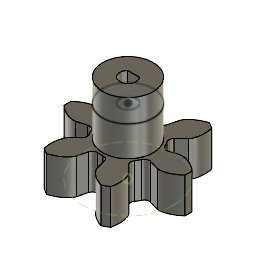
Motor Loading Gear (Autodesk Fusion 360 design; units mm, degrees)
part number: 2026-03-27-15-46-47-393
Autodesk Fusion 360 part; units mm, degrees
note: some values were not read from the file. Set by a fixed rule: which sketch regions a step uses.
(part 1 of 2)
sketch "Base Circle" plane through (0, 0, 0) normal (0, 0, 1) x (1, 0, 0)
  circle A0 centre (0, 0) radius 5.529
  circle A1 centre (0, 0) radius 1.75
  dimension "d28" = 3.5
  measures "d28" diameter of A1
extrude "Extrude1" add sketch "Base Circle" along normal blind 7 makes body 1
sketch "Gear Tooth" plane through (0, 0, 0) normal (0, 0, 1) x (1, 0, 0)
  spline S0 degree 5 poles (8.1355, -2.3104) (8.146, -2.3134) (8.1669, -2.3188) (8.1987, -2.3257) (8.2415, -2.3322) (8.2956, -2.3368) (8.3503, -2.3389) (8.4053, -2.3395) (8.4604, -2.3392) (8.5157, -2.3384) (8.5711, -2.3369) (8.6267, -2.3345) (8.6824, -2.3309) (8.7383, -2.3259) (8.7943, -2.3197) (8.8505, -2.3123) (8.9068, -2.3039) (8.9632, -2.2946) (9.0196, -2.2845) (9.0761, -2.2737) (9.1326, -2.2622) (9.1892, -2.2498) (9.2457, -2.2365) (9.3024, -2.2224) (9.359, -2.2074) (9.4157, -2.1917) (9.4723, -2.1751) (9.529, -2.1578) (9.5856, -2.1398) (9.6422, -2.1211) (9.6988, -2.1016) (9.7554, -2.0815) (9.8119, -2.0606) (9.8683, -2.0389) (9.9248, -2.0166) (9.9811, -1.9936) (10.0374, -1.9699) (10.0936, -1.9455) (10.1498, -1.9205) (10.2059, -1.8948) (10.2618, -1.8684) (10.3177, -1.8414) (10.3735, -1.8138) (10.4292, -1.7855) (10.4848, -1.7565) (10.5403, -1.7269) (10.5957, -1.6967) (10.6509, -1.6659) (10.706, -1.6345) (10.761, -1.6024) (10.8158, -1.5697) (10.8706, -1.5365) (10.9251, -1.5026) (10.9795, -1.4681) (11.0338, -1.4331) (11.0879, -1.3974) (11.1418, -1.3612) (11.1956, -1.3244) (11.2492, -1.287) (11.3026, -1.249) (11.3559, -1.2105) (11.4089, -1.1714) (11.4618, -1.1317) (11.5145, -1.0915) (11.567, -1.0507) (11.6193, -1.0094) (11.6713, -0.9676) (11.7232, -0.9251) (11.7749, -0.8822) (11.8263, -0.8387) (11.8775, -0.7947) (11.9183, -0.7591) (11.9488, -0.7321) (11.9691, -0.714) (11.9793, -0.705) knots 0 0 0 0 0 0 0.01428571 0.02857143 0.04285714 0.05714286 0.07142857 0.08571429 0.1 0.11428571 0.12857143 0.14285714 0.15714286 0.17142857 0.18571429 0.2 0.21428571 0.22857143 0.24285714 0.25714286 0.27142857 0.28571429 0.3 0.31428571 0.32857143 0.34285714 0.35714286 0.37142857 0.38571429 0.4 0.41428571 0.42857143 0.44285714 0.45714286 0.47142857 0.48571429 0.5 0.51428571 0.52857143 0.54285714 0.55714286 0.57142857 0.58571429 0.6 0.61428571 0.62857143 0.64285714 0.65714286 0.67142857 0.68571429 0.7 0.71428571 0.72857143 0.74285714 0.75714286 0.77142857 0.78571429 0.8 0.81428571 0.82857143 0.84285714 0.85714286 0.87142857 0.88571429 0.9 0.91428571 0.92857143 0.94285714 0.95714286 0.97142857 0.98571429 1 1 1 1 1 1
  spline S1 degree 5 poles (8.1355, 2.3104) (8.146, 2.3134) (8.1669, 2.3188) (8.1987, 2.3257) (8.2415, 2.3322) (8.2956, 2.3368) (8.3503, 2.3389) (8.4053, 2.3395) (8.4604, 2.3392) (8.5157, 2.3384) (8.5711, 2.3369) (8.6267, 2.3345) (8.6824, 2.3309) (8.7383, 2.3259) (8.7943, 2.3197) (8.8505, 2.3123) (8.9068, 2.3039) (8.9632, 2.2946) (9.0196, 2.2845) (9.0761, 2.2737) (9.1326, 2.2622) (9.1892, 2.2498) (9.2457, 2.2365) (9.3024, 2.2224) (9.359, 2.2074) (9.4157, 2.1917) (9.4723, 2.1751) (9.529, 2.1578) (9.5856, 2.1398) (9.6422, 2.1211) (9.6988, 2.1016) (9.7554, 2.0815) (9.8119, 2.0606) (9.8683, 2.0389) (9.9248, 2.0166) (9.9811, 1.9936) (10.0374, 1.9699) (10.0936, 1.9455) (10.1498, 1.9205) (10.2059, 1.8948) (10.2618, 1.8684) (10.3177, 1.8414) (10.3735, 1.8138) (10.4292, 1.7855) (10.4848, 1.7565) (10.5403, 1.7269) (10.5957, 1.6967) (10.6509, 1.6659) (10.706, 1.6345) (10.761, 1.6024) (10.8158, 1.5697) (10.8706, 1.5365) (10.9251, 1.5026) (10.9795, 1.4681) (11.0338, 1.4331) (11.0879, 1.3974) (11.1418, 1.3612) (11.1956, 1.3244) (11.2492, 1.287) (11.3026, 1.249) (11.3559, 1.2105) (11.4089, 1.1714) (11.4618, 1.1317) (11.5145, 1.0915) (11.567, 1.0507) (11.6193, 1.0094) (11.6713, 0.9676) (11.7232, 0.9251) (11.7749, 0.8822) (11.8263, 0.8387) (11.8775, 0.7947) (11.9183, 0.7591) (11.9488, 0.7321) (11.9691, 0.714) (11.9793, 0.705) knots 0 0 0 0 0 0 0.01428571 0.02857143 0.04285714 0.05714286 0.07142857 0.08571429 0.1 0.11428571 0.12857143 0.14285714 0.15714286 0.17142857 0.18571429 0.2 0.21428571 0.22857143 0.24285714 0.25714286 0.27142857 0.28571429 0.3 0.31428571 0.32857143 0.34285714 0.35714286 0.37142857 0.38571429 0.4 0.41428571 0.42857143 0.44285714 0.45714286 0.47142857 0.48571429 0.5 0.51428571 0.52857143 0.54285714 0.55714286 0.57142857 0.58571429 0.6 0.61428571 0.62857143 0.64285714 0.65714286 0.67142857 0.68571429 0.7 0.71428571 0.72857143 0.74285714 0.75714286 0.77142857 0.78571429 0.8 0.81428571 0.82857143 0.84285714 0.85714286 0.87142857 0.88571429 0.9 0.91428571 0.92857143 0.94285714 0.95714286 0.97142857 0.98571429 1 1 1 1 1 1
  arc A0 (11.9793, -0.705) -> (11.9793, 0.705) centre (0, 0) ccw
  line L0 (5.3091, -1.5077) -> (8.1355, -2.3104)
  line L1 (5.3091, 1.5077) -> (8.1355, 2.3104)
  line L2 (5.3091, -1.5077) -> (5.3091, 1.5077)
  point P0 (8.3903, -2.3392)
  point P1 (8.6545, -2.3325)
  point P2 (8.9246, -2.3008)
  point P3 (9.1989, -2.2473)
  point P4 (9.4764, -2.1737)
  point P5 (9.7561, -2.081)
  point P6 (10.0371, -1.9699)
  point P7 (10.3188, -1.8408)
  point P8 (10.6002, -1.694)
  point P9 (10.8807, -1.53)
  point P10 (11.1596, -1.3489)
  point P11 (11.4361, -1.1509)
  point P12 (11.7096, -0.9362)
  point P13 (8.3903, 2.3392)
  point P14 (8.6545, 2.3325)
  point P15 (8.9246, 2.3008)
  point P16 (9.1989, 2.2473)
  point P17 (9.4764, 2.1737)
  point P18 (9.7561, 2.081)
  point P19 (10.0371, 1.9699)
  point P20 (10.3188, 1.8408)
  point P21 (10.6002, 1.694)
  point P22 (10.8807, 1.53)
  point P23 (11.1596, 1.3489)
  point P24 (11.4361, 1.1509)
  point P25 (11.7096, 0.9362)
extrude "Extrude2" add sketch "Gear Tooth" along normal blind 7 bodies 1
fillet "Fillet1" radius 1 2 edges at (5.3187, -1.5104, 3.5) (5.3187, 1.5104, 3.5) on bodies 1
pattern_circular "C-Pattern1" count 6 over 360 about axis through (0, 0, 0) along (0, 0, 1) of "Extrude2", "Fillet1"
sketch "Diametrial Pitch Circle" plane through (0, 0, 0) normal (0, 0, 1) x (1, 0, 0)
  circle A0 centre (0, 0) radius 9 construction
sketch "Sketch4" plane through (0, 0, 7) normal (0, 0, 1) x (-1, 0, 0)
  arc A0 (-4.5104, 3.1978) -> (-5.0246, 2.3072) centre (0, 0) ccw
  arc A1 (-6.2065, 1.7626) -> (-5.0246, 2.3072) centre (-5.9334, 2.7245) ccw
  line L0 (-6.2065, 1.7626) -> (-8.1355, 2.3104)
  line L1 (-8.1355, -2.3104) -> (-6.2065, -1.7626)
  arc A2 (-5.0246, -2.3072) -> (-6.2065, -1.7626) centre (-5.9334, -2.7245) ccw
  line L2 (-4.6297, -4.4937) -> (-6.0686, -5.8904)
  line L3 (-2.0669, -8.2008) -> (-1.5768, -6.2563)
  line L4 (1.5768, -6.2563) -> (2.0669, -8.2008)
  line L5 (6.0686, -5.8904) -> (4.6297, -4.4937)
  line L6 (6.2065, -1.7626) -> (8.1355, -2.3104)
  line L7 (8.1355, 2.3104) -> (6.2065, 1.7626)
  line L8 (4.6297, 4.4937) -> (6.0686, 5.8904)
  line L9 (2.0669, 8.2008) -> (1.5768, 6.2563)
  line L10 (-1.5768, 6.2563) -> (-2.0669, 8.2008)
  line L11 (-6.0686, 5.8904) -> (-4.6297, 4.4937)
  circle A3 centre (0, 0) radius 1.75
  circle A4 centre (0, 0) radius 3.5
  circle A5 centre (0, 0) radius 5
  arc A6 (-4.6297, -4.4937) -> (-4.5104, -3.1978) centre (-5.3262, -3.7762) ccw
  arc A7 (-0.5142, -5.505) -> (-1.5768, -6.2563) centre (-0.6071, -6.5007) ccw
  arc A8 (1.5768, -6.2563) -> (0.5142, -5.505) centre (0.6071, -6.5007) ccw
  arc A9 (4.5104, -3.1978) -> (4.6297, -4.4937) centre (5.3262, -3.7762) ccw
  arc A10 (6.2065, -1.7626) -> (5.0246, -2.3072) centre (5.9334, -2.7245) ccw
  arc A11 (5.0246, 2.3072) -> (6.2065, 1.7626) centre (5.9334, 2.7245) ccw
  arc A12 (4.6297, 4.4937) -> (4.5104, 3.1978) centre (5.3262, 3.7762) ccw
  arc A13 (0.5142, 5.505) -> (1.5768, 6.2563) centre (0.6071, 6.5007) ccw
  arc A14 (-1.5768, 6.2563) -> (-0.5142, 5.505) centre (-0.6071, 6.5007) ccw
  arc A15 (-4.5104, 3.1978) -> (-4.6297, 4.4937) centre (-5.3262, 3.7762) ccw
  spline S0 degree 5 poles (-8.1355, 2.3104) (-8.146, 2.3134) (-8.1669, 2.3188) (-8.1987, 2.3257) (-8.2415, 2.3322) (-8.2956, 2.3368) (-8.3503, 2.3389) (-8.4053, 2.3395) (-8.4604, 2.3392) (-8.5157, 2.3384) (-8.5711, 2.3369) (-8.6267, 2.3345) (-8.6824, 2.3309) (-8.7383, 2.3259) (-8.7943, 2.3197) (-8.8505, 2.3123) (-8.9068, 2.3039) (-8.9632, 2.2946) (-9.0196, 2.2845) (-9.0761, 2.2737) (-9.1326, 2.2622) (-9.1892, 2.2498) (-9.2457, 2.2365) (-9.3024, 2.2224) (-9.359, 2.2074) (-9.4157, 2.1917) (-9.4723, 2.1751) (-9.529, 2.1578) (-9.5856, 2.1398) (-9.6422, 2.1211) (-9.6988, 2.1016) (-9.7554, 2.0815) (-9.8119, 2.0606) (-9.8683, 2.0389) (-9.9248, 2.0166) (-9.9811, 1.9936) (-10.0374, 1.9699) (-10.0936, 1.9455) (-10.1498, 1.9205) (-10.2059, 1.8948) (-10.2618, 1.8684) (-10.3177, 1.8414) (-10.3735, 1.8138) (-10.4292, 1.7855) (-10.4848, 1.7565) (-10.5403, 1.7269) (-10.5957, 1.6967) (-10.6509, 1.6659) (-10.706, 1.6345) (-10.761, 1.6024) (-10.8158, 1.5697) (-10.8706, 1.5365) (-10.9251, 1.5026) (-10.9795, 1.4681) (-11.0338, 1.4331) (-11.0879, 1.3974) (-11.1418, 1.3612) (-11.1956, 1.3244) (-11.2492, 1.287) (-11.3026, 1.249) (-11.3559, 1.2105) (-11.4089, 1.1714) (-11.4618, 1.1317) (-11.5145, 1.0915) (-11.567, 1.0507) (-11.6193, 1.0094) (-11.6713, 0.9676) (-11.7232, 0.9251) (-11.7749, 0.8822) (-11.8263, 0.8387) (-11.8775, 0.7947) (-11.9183, 0.7591) (-11.9488, 0.7321) (-11.9691, 0.714) (-11.9793, 0.705) knots 0 0 0 0 0 0 0.01428571 0.02857143 0.04285714 0.05714286 0.07142857 0.08571429 0.1 0.11428571 0.12857143 0.14285714 0.15714286 0.17142857 0.18571429 0.2 0.21428571 0.22857143 0.24285714 0.25714286 0.27142857 0.28571429 0.3 0.31428571 0.32857143 0.34285714 0.35714286 0.37142857 0.38571429 0.4 0.41428571 0.42857143 0.44285714 0.45714286 0.47142857 0.48571429 0.5 0.51428571 0.52857143 0.54285714 0.55714286 0.57142857 0.58571429 0.6 0.61428571 0.62857143 0.64285714 0.65714286 0.67142857 0.68571429 0.7 0.71428571 0.72857143 0.74285714 0.75714286 0.77142857 0.78571429 0.8 0.81428571 0.82857143 0.84285714 0.85714286 0.87142857 0.88571429 0.9 0.91428571 0.92857143 0.94285714 0.95714286 0.97142857 0.98571429 1 1 1 1 1 1
  arc A16 (-11.9793, 0.705) -> (-11.9793, -0.705) centre (0, 0) ccw
  spline S1 degree 5 poles (-11.9793, -0.705) (-11.9691, -0.714) (-11.9488, -0.7321) (-11.9183, -0.7591) (-11.8775, -0.7947) (-11.8263, -0.8387) (-11.7749, -0.8822) (-11.7232, -0.9251) (-11.6713, -0.9676) (-11.6193, -1.0094) (-11.567, -1.0507) (-11.5145, -1.0915) (-11.4618, -1.1317) (-11.4089, -1.1714) (-11.3559, -1.2105) (-11.3026, -1.249) (-11.2492, -1.287) (-11.1956, -1.3244) (-11.1418, -1.3612) (-11.0879, -1.3974) (-11.0338, -1.4331) (-10.9795, -1.4681) (-10.9251, -1.5026) (-10.8706, -1.5365) (-10.8158, -1.5697) (-10.761, -1.6024) (-10.706, -1.6345) (-10.6509, -1.6659) (-10.5957, -1.6967) (-10.5403, -1.7269) (-10.4848, -1.7565) (-10.4292, -1.7855) (-10.3735, -1.8138) (-10.3177, -1.8414) (-10.2618, -1.8684) (-10.2059, -1.8948) (-10.1498, -1.9205) (-10.0936, -1.9455) (-10.0374, -1.9699) (-9.9811, -1.9936) (-9.9248, -2.0166) (-9.8683, -2.0389) (-9.8119, -2.0606) (-9.7554, -2.0815) (-9.6988, -2.1016) (-9.6422, -2.1211) (-9.5856, -2.1398) (-9.529, -2.1578) (-9.4723, -2.1751) (-9.4157, -2.1917) (-9.359, -2.2074) (-9.3024, -2.2224) (-9.2457, -2.2365) (-9.1892, -2.2498) (-9.1326, -2.2622) (-9.0761, -2.2737) (-9.0196, -2.2845) (-8.9632, -2.2946) (-8.9068, -2.3039) (-8.8505, -2.3123) (-8.7943, -2.3197) (-8.7383, -2.3259) (-8.6824, -2.3309) (-8.6267, -2.3345) (-8.5711, -2.3369) (-8.5157, -2.3384) (-8.4604, -2.3392) (-8.4053, -2.3395) (-8.3503, -2.3389) (-8.2956, -2.3368) (-8.2415, -2.3322) (-8.1987, -2.3257) (-8.1669, -2.3188) (-8.146, -2.3134) (-8.1355, -2.3104) knots -1 -1 -1 -1 -1 -1 -0.98571429 -0.97142857 -0.95714286 -0.94285714 -0.92857143 -0.91428571 -0.9 -0.88571429 -0.87142857 -0.85714286 -0.84285714 -0.82857143 -0.81428571 -0.8 -0.78571429 -0.77142857 -0.75714286 -0.74285714 -0.72857143 -0.71428571 -0.7 -0.68571429 -0.67142857 -0.65714286 -0.64285714 -0.62857143 -0.61428571 -0.6 -0.58571429 -0.57142857 -0.55714286 -0.54285714 -0.52857143 -0.51428571 -0.5 -0.48571429 -0.47142857 -0.45714286 -0.44285714 -0.42857143 -0.41428571 -0.4 -0.38571429 -0.37142857 -0.35714286 -0.34285714 -0.32857143 -0.31428571 -0.3 -0.28571429 -0.27142857 -0.25714286 -0.24285714 -0.22857143 -0.21428571 -0.2 -0.18571429 -0.17142857 -0.15714286 -0.14285714 -0.12857143 -0.11428571 -0.1 -0.08571429 -0.07142857 -0.05714286 -0.04285714 -0.02857143 -0.01428571 0 0 0 0 0 0
  arc A17 (-5.0246, -2.3072) -> (-4.5104, -3.1978) centre (0, 0) ccw
  spline S2 degree 5 poles (-6.0686, -5.8904) (-6.0764, -5.8979) (-6.0916, -5.9134) (-6.1134, -5.9374) (-6.1405, -5.9712) (-6.1715, -6.0158) (-6.2007, -6.0621) (-6.2287, -6.1095) (-6.2561, -6.1573) (-6.283, -6.2056) (-6.3094, -6.2544) (-6.3351, -6.3037) (-6.3598, -6.3537) (-6.3835, -6.4046) (-6.4061, -6.4563) (-6.4278, -6.5086) (-6.4486, -6.5616) (-6.4688, -6.6151) (-6.4883, -6.669) (-6.5072, -6.7233) (-6.5254, -6.778) (-6.5429, -6.8332) (-6.5597, -6.8888) (-6.5758, -6.9449) (-6.5912, -7.0014) (-6.6059, -7.0584) (-6.6199, -7.1157) (-6.6332, -7.1734) (-6.6459, -7.2315) (-6.658, -7.2899) (-6.6695, -7.3486) (-6.6803, -7.4077) (-6.6904, -7.467) (-6.6999, -7.5268) (-6.7088, -7.5868) (-6.7171, -7.6471) (-6.7247, -7.7077) (-6.7317, -7.7686) (-6.7381, -7.8297) (-6.7439, -7.8911) (-6.749, -7.9528) (-6.7536, -8.0147) (-6.7575, -8.0769) (-6.7609, -8.1392) (-6.7636, -8.2019) (-6.7657, -8.2647) (-6.7672, -8.3277) (-6.7682, -8.391) (-6.7685, -8.4545) (-6.7682, -8.5181) (-6.7674, -8.5819) (-6.7659, -8.6459) (-6.7638, -8.7101) (-6.7612, -8.7745) (-6.758, -8.839) (-6.7541, -8.9037) (-6.7497, -8.9685) (-6.7447, -9.0335) (-6.7391, -9.0986) (-6.733, -9.1639) (-6.7262, -9.2292) (-6.7189, -9.2947) (-6.711, -9.3604) (-6.7025, -9.4261) (-6.6935, -9.4919) (-6.6838, -9.5579) (-6.6736, -9.6239) (-6.6628, -9.69) (-6.6514, -9.7562) (-6.6395, -9.8225) (-6.627, -9.8889) (-6.6165, -9.942) (-6.6084, -9.9819) (-6.6029, -10.0086) (-6.6001, -10.0219) knots 0 0 0 0 0 0 0.01428571 0.02857143 0.04285714 0.05714286 0.07142857 0.08571429 0.1 0.11428571 0.12857143 0.14285714 0.15714286 0.17142857 0.18571429 0.2 0.21428571 0.22857143 0.24285714 0.25714286 0.27142857 0.28571429 0.3 0.31428571 0.32857143 0.34285714 0.35714286 0.37142857 0.38571429 0.4 0.41428571 0.42857143 0.44285714 0.45714286 0.47142857 0.48571429 0.5 0.51428571 0.52857143 0.54285714 0.55714286 0.57142857 0.58571429 0.6 0.61428571 0.62857143 0.64285714 0.65714286 0.67142857 0.68571429 0.7 0.71428571 0.72857143 0.74285714 0.75714286 0.77142857 0.78571429 0.8 0.81428571 0.82857143 0.84285714 0.85714286 0.87142857 0.88571429 0.9 0.91428571 0.92857143 0.94285714 0.95714286 0.97142857 0.98571429 1 1 1 1 1 1
  arc A18 (-6.6001, -10.0219) -> (-5.3791, -10.7268) centre (0, 0) ccw
  spline S3 degree 5 poles (-5.3791, -10.7268) (-5.3662, -10.7226) (-5.3404, -10.7141) (-5.3018, -10.7011) (-5.2505, -10.6836) (-5.1868, -10.6612) (-5.1234, -10.6384) (-5.0604, -10.6152) (-4.9977, -10.5915) (-4.9354, -10.5673) (-4.8735, -10.5427) (-4.812, -10.5176) (-4.7508, -10.4921) (-4.69, -10.4661) (-4.6296, -10.4397) (-4.5696, -10.4129) (-4.5101, -10.3856) (-4.4509, -10.3578) (-4.3921, -10.3297) (-4.3338, -10.3011) (-4.2758, -10.2721) (-4.2183, -10.2426) (-4.1613, -10.2127) (-4.1047, -10.1824) (-4.0485, -10.1517) (-3.9928, -10.1205) (-3.9375, -10.0889) (-3.8827, -10.0569) (-3.8284, -10.0245) (-3.7746, -9.9916) (-3.7212, -9.9584) (-3.6684, -9.9247) (-3.616, -9.8906) (-3.5641, -9.8561) (-3.5128, -9.8212) (-3.462, -9.7859) (-3.4117, -9.7502) (-3.3619, -9.7141) (-3.3127, -9.6776) (-3.264, -9.6407) (-3.2159, -9.6034) (-3.1684, -9.5657) (-3.1214, -9.5276) (-3.0751, -9.4891) (-3.0293, -9.4502) (-2.9842, -9.4109) (-2.9397, -9.3713) (-2.8958, -9.3312) (-2.8525, -9.2908) (-2.8098, -9.25) (-2.7678, -9.2089) (-2.7265, -9.1673) (-2.686, -9.1253) (-2.6462, -9.0829) (-2.6072, -9.0401) (-2.5689, -8.997) (-2.5313, -8.9535) (-2.4944, -8.9097) (-2.4582, -8.8655) (-2.4228, -8.8209) (-2.3882, -8.776) (-2.3548, -8.7305) (-2.3226, -8.6846) (-2.2916, -8.6382) (-2.2617, -8.5913) (-2.2327, -8.544) (-2.2044, -8.4966) (-2.1766, -8.4489) (-2.1496, -8.401) (-2.1241, -8.3526) (-2.101, -8.3034) (-2.0852, -8.2631) (-2.0753, -8.2322) (-2.0696, -8.2113) (-2.0669, -8.2008) knots -1 -1 -1 -1 -1 -1 -0.98571429 -0.97142857 -0.95714286 -0.94285714 -0.92857143 -0.91428571 -0.9 -0.88571429 -0.87142857 -0.85714286 -0.84285714 -0.82857143 -0.81428571 -0.8 -0.78571429 -0.77142857 -0.75714286 -0.74285714 -0.72857143 -0.71428571 -0.7 -0.68571429 -0.67142857 -0.65714286 -0.64285714 -0.62857143 -0.61428571 -0.6 -0.58571429 -0.57142857 -0.55714286 -0.54285714 -0.52857143 -0.51428571 -0.5 -0.48571429 -0.47142857 -0.45714286 -0.44285714 -0.42857143 -0.41428571 -0.4 -0.38571429 -0.37142857 -0.35714286 -0.34285714 -0.32857143 -0.31428571 -0.3 -0.28571429 -0.27142857 -0.25714286 -0.24285714 -0.22857143 -0.21428571 -0.2 -0.18571429 -0.17142857 -0.15714286 -0.14285714 -0.12857143 -0.11428571 -0.1 -0.08571429 -0.07142857 -0.05714286 -0.04285714 -0.02857143 -0.01428571 0 0 0 0 0 0
  arc A19 (-0.5142, -5.505) -> (0.5142, -5.505) centre (0, 0) ccw
  spline S4 degree 5 poles (2.0669, -8.2008) (2.0696, -8.2113) (2.0753, -8.2322) (2.0852, -8.2631) (2.101, -8.3034) (2.1241, -8.3526) (2.1496, -8.401) (2.1766, -8.4489) (2.2044, -8.4966) (2.2327, -8.544) (2.2617, -8.5913) (2.2916, -8.6382) (2.3226, -8.6846) (2.3548, -8.7305) (2.3882, -8.776) (2.4228, -8.8209) (2.4582, -8.8655) (2.4944, -8.9097) (2.5313, -8.9535) (2.5689, -8.997) (2.6072, -9.0401) (2.6462, -9.0829) (2.686, -9.1253) (2.7265, -9.1673) (2.7678, -9.2089) (2.8098, -9.25) (2.8525, -9.2908) (2.8958, -9.3312) (2.9397, -9.3713) (2.9842, -9.4109) (3.0293, -9.4502) (3.0751, -9.4891) (3.1214, -9.5276) (3.1684, -9.5657) (3.2159, -9.6034) (3.264, -9.6407) (3.3127, -9.6776) (3.3619, -9.7141) (3.4117, -9.7502) (3.462, -9.7859) (3.5128, -9.8212) (3.5641, -9.8561) (3.616, -9.8906) (3.6684, -9.9247) (3.7212, -9.9584) (3.7746, -9.9916) (3.8284, -10.0245) (3.8827, -10.0569) (3.9375, -10.0889) (3.9928, -10.1205) (4.0485, -10.1517) (4.1047, -10.1824) (4.1613, -10.2127) (4.2183, -10.2426) (4.2758, -10.2721) (4.3338, -10.3011) (4.3921, -10.3297) (4.4509, -10.3578) (4.5101, -10.3856) (4.5696, -10.4129) (4.6296, -10.4397) (4.69, -10.4661) (4.7508, -10.4921) (4.812, -10.5176) (4.8735, -10.5427) (4.9354, -10.5673) (4.9977, -10.5915) (5.0604, -10.6152) (5.1234, -10.6384) (5.1868, -10.6612) (5.2505, -10.6836) (5.3018, -10.7011) (5.3404, -10.7141) (5.3662, -10.7226) (5.3791, -10.7268) knots 0 0 0 0 0 0 0.01428571 0.02857143 0.04285714 0.05714286 0.07142857 0.08571429 0.1 0.11428571 0.12857143 0.14285714 0.15714286 0.17142857 0.18571429 0.2 0.21428571 0.22857143 0.24285714 0.25714286 0.27142857 0.28571429 0.3 0.31428571 0.32857143 0.34285714 0.35714286 0.37142857 0.38571429 0.4 0.41428571 0.42857143 0.44285714 0.45714286 0.47142857 0.48571429 0.5 0.51428571 0.52857143 0.54285714 0.55714286 0.57142857 0.58571429 0.6 0.61428571 0.62857143 0.64285714 0.65714286 0.67142857 0.68571429 0.7 0.71428571 0.72857143 0.74285714 0.75714286 0.77142857 0.78571429 0.8 0.81428571 0.82857143 0.84285714 0.85714286 0.87142857 0.88571429 0.9 0.91428571 0.92857143 0.94285714 0.95714286 0.97142857 0.98571429 1 1 1 1 1 1
  arc A20 (5.3791, -10.7268) -> (6.6001, -10.0219) centre (0, 0) ccw
  spline S5 degree 5 poles (6.6001, -10.0219) (6.6029, -10.0086) (6.6084, -9.9819) (6.6165, -9.942) (6.627, -9.8889) (6.6395, -9.8225) (6.6514, -9.7562) (6.6628, -9.69) (6.6736, -9.6239) (6.6838, -9.5579) (6.6935, -9.4919) (6.7025, -9.4261) (6.711, -9.3604) (6.7189, -9.2947) (6.7262, -9.2292) (6.733, -9.1639) (6.7391, -9.0986) (6.7447, -9.0335) (6.7497, -8.9685) (6.7541, -8.9037) (6.758, -8.839) (6.7612, -8.7745) (6.7638, -8.7101) (6.7659, -8.6459) (6.7674, -8.5819) (6.7682, -8.5181) (6.7685, -8.4545) (6.7682, -8.391) (6.7672, -8.3277) (6.7657, -8.2647) (6.7636, -8.2019) (6.7609, -8.1392) (6.7575, -8.0769) (6.7536, -8.0147) (6.749, -7.9528) (6.7439, -7.8911) (6.7381, -7.8297) (6.7317, -7.7686) (6.7247, -7.7077) (6.7171, -7.6471) (6.7088, -7.5868) (6.6999, -7.5268) (6.6904, -7.467) (6.6803, -7.4077) (6.6695, -7.3486) (6.658, -7.2899) (6.6459, -7.2315) (6.6332, -7.1734) (6.6199, -7.1157) (6.6059, -7.0584) (6.5912, -7.0014) (6.5758, -6.9449) (6.5597, -6.8888) (6.5429, -6.8332) (6.5254, -6.778) (6.5072, -6.7233) (6.4883, -6.669) (6.4688, -6.6151) (6.4486, -6.5616) (6.4278, -6.5086) (6.4061, -6.4563) (6.3835, -6.4046) (6.3598, -6.3537) (6.3351, -6.3037) (6.3094, -6.2544) (6.283, -6.2056) (6.2561, -6.1573) (6.2287, -6.1095) (6.2007, -6.0621) (6.1715, -6.0158) (6.1405, -5.9712) (6.1134, -5.9374) (6.0916, -5.9134) (6.0764, -5.8979) (6.0686, -5.8904) knots -1 -1 -1 -1 -1 -1 -0.98571429 -0.97142857 -0.95714286 -0.94285714 -0.92857143 -0.91428571 -0.9 -0.88571429 -0.87142857 -0.85714286 -0.84285714 -0.82857143 -0.81428571 -0.8 -0.78571429 -0.77142857 -0.75714286 -0.74285714 -0.72857143 -0.71428571 -0.7 -0.68571429 -0.67142857 -0.65714286 -0.64285714 -0.62857143 -0.61428571 -0.6 -0.58571429 -0.57142857 -0.55714286 -0.54285714 -0.52857143 -0.51428571 -0.5 -0.48571429 -0.47142857 -0.45714286 -0.44285714 -0.42857143 -0.41428571 -0.4 -0.38571429 -0.37142857 -0.35714286 -0.34285714 -0.32857143 -0.31428571 -0.3 -0.28571429 -0.27142857 -0.25714286 -0.24285714 -0.22857143 -0.21428571 -0.2 -0.18571429 -0.17142857 -0.15714286 -0.14285714 -0.12857143 -0.11428571 -0.1 -0.08571429 -0.07142857 -0.05714286 -0.04285714 -0.02857143 -0.01428571 0 0 0 0 0 0
  arc A21 (4.5104, -3.1978) -> (5.0246, -2.3072) centre (0, 0) ccw
  spline S6 degree 5 poles (8.1355, -2.3104) (8.146, -2.3134) (8.1669, -2.3188) (8.1987, -2.3257) (8.2415, -2.3322) (8.2956, -2.3368) (8.3503, -2.3389) (8.4053, -2.3395) (8.4604, -2.3392) (8.5157, -2.3384) (8.5711, -2.3369) (8.6267, -2.3345) (8.6824, -2.3309) (8.7383, -2.3259) (8.7943, -2.3197) (8.8505, -2.3123) (8.9068, -2.3039) (8.9632, -2.2946) (9.0196, -2.2845) (9.0761, -2.2737) (9.1326, -2.2622) (9.1892, -2.2498) (9.2457, -2.2365) (9.3024, -2.2224) (9.359, -2.2074) (9.4157, -2.1917) (9.4723, -2.1751) (9.529, -2.1578) (9.5856, -2.1398) (9.6422, -2.1211) (9.6988, -2.1016) (9.7554, -2.0815) (9.8119, -2.0606) (9.8683, -2.0389) (9.9248, -2.0166) (9.9811, -1.9936) (10.0374, -1.9699) (10.0936, -1.9455) (10.1498, -1.9205) (10.2059, -1.8948) (10.2618, -1.8684) (10.3177, -1.8414) (10.3735, -1.8138) (10.4292, -1.7855) (10.4848, -1.7565) (10.5403, -1.7269) (10.5957, -1.6967) (10.6509, -1.6659) (10.706, -1.6345) (10.761, -1.6024) (10.8158, -1.5697) (10.8706, -1.5365) (10.9251, -1.5026) (10.9795, -1.4681) (11.0338, -1.4331) (11.0879, -1.3974) (11.1418, -1.3612) (11.1956, -1.3244) (11.2492, -1.287) (11.3026, -1.249) (11.3559, -1.2105) (11.4089, -1.1714) (11.4618, -1.1317) (11.5145, -1.0915) (11.567, -1.0507) (11.6193, -1.0094) (11.6713, -0.9676) (11.7232, -0.9251) (11.7749, -0.8822) (11.8263, -0.8387) (11.8775, -0.7947) (11.9183, -0.7591) (11.9488, -0.7321) (11.9691, -0.714) (11.9793, -0.705) knots 0 0 0 0 0 0 0.01428571 0.02857143 0.04285714 0.05714286 0.07142857 0.08571429 0.1 0.11428571 0.12857143 0.14285714 0.15714286 0.17142857 0.18571429 0.2 0.21428571 0.22857143 0.24285714 0.25714286 0.27142857 0.28571429 0.3 0.31428571 0.32857143 0.34285714 0.35714286 0.37142857 0.38571429 0.4 0.41428571 0.42857143 0.44285714 0.45714286 0.47142857 0.48571429 0.5 0.51428571 0.52857143 0.54285714 0.55714286 0.57142857 0.58571429 0.6 0.61428571 0.62857143 0.64285714 0.65714286 0.67142857 0.68571429 0.7 0.71428571 0.72857143 0.74285714 0.75714286 0.77142857 0.78571429 0.8 0.81428571 0.82857143 0.84285714 0.85714286 0.87142857 0.88571429 0.9 0.91428571 0.92857143 0.94285714 0.95714286 0.97142857 0.98571429 1 1 1 1 1 1
  arc A22 (11.9793, -0.705) -> (11.9793, 0.705) centre (0, 0) ccw
  spline S7 degree 5 poles (11.9793, 0.705) (11.9691, 0.714) (11.9488, 0.7321) (11.9183, 0.7591) (11.8775, 0.7947) (11.8263, 0.8387) (11.7749, 0.8822) (11.7232, 0.9251) (11.6713, 0.9676) (11.6193, 1.0094) (11.567, 1.0507) (11.5145, 1.0915) (11.4618, 1.1317) (11.4089, 1.1714) (11.3559, 1.2105) (11.3026, 1.249) (11.2492, 1.287) (11.1956, 1.3244) (11.1418, 1.3612) (11.0879, 1.3974) (11.0338, 1.4331) (10.9795, 1.4681) (10.9251, 1.5026) (10.8706, 1.5365) (10.8158, 1.5697) (10.761, 1.6024) (10.706, 1.6345) (10.6509, 1.6659) (10.5957, 1.6967) (10.5403, 1.7269) (10.4848, 1.7565) (10.4292, 1.7855) (10.3735, 1.8138) (10.3177, 1.8414) (10.2618, 1.8684) (10.2059, 1.8948) (10.1498, 1.9205) (10.0936, 1.9455) (10.0374, 1.9699) (9.9811, 1.9936) (9.9248, 2.0166) (9.8683, 2.0389) (9.8119, 2.0606) (9.7554, 2.0815) (9.6988, 2.1016) (9.6422, 2.1211) (9.5856, 2.1398) (9.529, 2.1578) (9.4723, 2.1751) (9.4157, 2.1917) (9.359, 2.2074) (9.3024, 2.2224) (9.2457, 2.2365) (9.1892, 2.2498) (9.1326, 2.2622) (9.0761, 2.2737) (9.0196, 2.2845) (8.9632, 2.2946) (8.9068, 2.3039) (8.8505, 2.3123) (8.7943, 2.3197) (8.7383, 2.3259) (8.6824, 2.3309) (8.6267, 2.3345) (8.5711, 2.3369) (8.5157, 2.3384) (8.4604, 2.3392) (8.4053, 2.3395) (8.3503, 2.3389) (8.2956, 2.3368) (8.2415, 2.3322) (8.1987, 2.3257) (8.1669, 2.3188) (8.146, 2.3134) (8.1355, 2.3104) knots -1 -1 -1 -1 -1 -1 -0.98571429 -0.97142857 -0.95714286 -0.94285714 -0.92857143 -0.91428571 -0.9 -0.88571429 -0.87142857 -0.85714286 -0.84285714 -0.82857143 -0.81428571 -0.8 -0.78571429 -0.77142857 -0.75714286 -0.74285714 -0.72857143 -0.71428571 -0.7 -0.68571429 -0.67142857 -0.65714286 -0.64285714 -0.62857143 -0.61428571 -0.6 -0.58571429 -0.57142857 -0.55714286 -0.54285714 -0.52857143 -0.51428571 -0.5 -0.48571429 -0.47142857 -0.45714286 -0.44285714 -0.42857143 -0.41428571 -0.4 -0.38571429 -0.37142857 -0.35714286 -0.34285714 -0.32857143 -0.31428571 -0.3 -0.28571429 -0.27142857 -0.25714286 -0.24285714 -0.22857143 -0.21428571 -0.2 -0.18571429 -0.17142857 -0.15714286 -0.14285714 -0.12857143 -0.11428571 -0.1 -0.08571429 -0.07142857 -0.05714286 -0.04285714 -0.02857143 -0.01428571 0 0 0 0 0 0
  arc A23 (5.0246, 2.3072) -> (4.5104, 3.1978) centre (0, 0) ccw
  spline S8 degree 5 poles (6.0686, 5.8904) (6.0764, 5.8979) (6.0916, 5.9134) (6.1134, 5.9374) (6.1405, 5.9712) (6.1715, 6.0158) (6.2007, 6.0621) (6.2287, 6.1095) (6.2561, 6.1573) (6.283, 6.2056) (6.3094, 6.2544) (6.3351, 6.3037) (6.3598, 6.3537) (6.3835, 6.4046) (6.4061, 6.4563) (6.4278, 6.5086) (6.4486, 6.5616) (6.4688, 6.6151) (6.4883, 6.669) (6.5072, 6.7233) (6.5254, 6.778) (6.5429, 6.8332) (6.5597, 6.8888) (6.5758, 6.9449) (6.5912, 7.0014) (6.6059, 7.0584) (6.6199, 7.1157) (6.6332, 7.1734) (6.6459, 7.2315) (6.658, 7.2899) (6.6695, 7.3486) (6.6803, 7.4077) (6.6904, 7.467) (6.6999, 7.5268) (6.7088, 7.5868) (6.7171, 7.6471) (6.7247, 7.7077) (6.7317, 7.7686) (6.7381, 7.8297) (6.7439, 7.8911) (6.749, 7.9528) (6.7536, 8.0147) (6.7575, 8.0769) (6.7609, 8.1392) (6.7636, 8.2019) (6.7657, 8.2647) (6.7672, 8.3277) (6.7682, 8.391) (6.7685, 8.4545) (6.7682, 8.5181) (6.7674, 8.5819) (6.7659, 8.6459) (6.7638, 8.7101) (6.7612, 8.7745) (6.758, 8.839) (6.7541, 8.9037) (6.7497, 8.9685) (6.7447, 9.0335) (6.7391, 9.0986) (6.733, 9.1639) (6.7262, 9.2292) (6.7189, 9.2947) (6.711, 9.3604) (6.7025, 9.4261) (6.6935, 9.4919) (6.6838, 9.5579) (6.6736, 9.6239) (6.6628, 9.69) (6.6514, 9.7562) (6.6395, 9.8225) (6.627, 9.8889) (6.6165, 9.942) (6.6084, 9.9819) (6.6029, 10.0086) (6.6001, 10.0219) knots 0 0 0 0 0 0 0.01428571 0.02857143 0.04285714 0.05714286 0.07142857 0.08571429 0.1 0.11428571 0.12857143 0.14285714 0.15714286 0.17142857 0.18571429 0.2 0.21428571 0.22857143 0.24285714 0.25714286 0.27142857 0.28571429 0.3 0.31428571 0.32857143 0.34285714 0.35714286 0.37142857 0.38571429 0.4 0.41428571 0.42857143 0.44285714 0.45714286 0.47142857 0.48571429 0.5 0.51428571 0.52857143 0.54285714 0.55714286 0.57142857 0.58571429 0.6 0.61428571 0.62857143 0.64285714 0.65714286 0.67142857 0.68571429 0.7 0.71428571 0.72857143 0.74285714 0.75714286 0.77142857 0.78571429 0.8 0.81428571 0.82857143 0.84285714 0.85714286 0.87142857 0.88571429 0.9 0.91428571 0.92857143 0.94285714 0.95714286 0.97142857 0.98571429 1 1 1 1 1 1
  arc A24 (6.6001, 10.0219) -> (5.3791, 10.7268) centre (0, 0) ccw
  spline S9 degree 5 poles (5.3791, 10.7268) (5.3662, 10.7226) (5.3404, 10.7141) (5.3018, 10.7011) (5.2505, 10.6836) (5.1868, 10.6612) (5.1234, 10.6384) (5.0604, 10.6152) (4.9977, 10.5915) (4.9354, 10.5673) (4.8735, 10.5427) (4.812, 10.5176) (4.7508, 10.4921) (4.69, 10.4661) (4.6296, 10.4397) (4.5696, 10.4129) (4.5101, 10.3856) (4.4509, 10.3578) (4.3921, 10.3297) (4.3338, 10.3011) (4.2758, 10.2721) (4.2183, 10.2426) (4.1613, 10.2127) (4.1047, 10.1824) (4.0485, 10.1517) (3.9928, 10.1205) (3.9375, 10.0889) (3.8827, 10.0569) (3.8284, 10.0245) (3.7746, 9.9916) (3.7212, 9.9584) (3.6684, 9.9247) (3.616, 9.8906) (3.5641, 9.8561) (3.5128, 9.8212) (3.462, 9.7859) (3.4117, 9.7502) (3.3619, 9.7141) (3.3127, 9.6776) (3.264, 9.6407) (3.2159, 9.6034) (3.1684, 9.5657) (3.1214, 9.5276) (3.0751, 9.4891) (3.0293, 9.4502) (2.9842, 9.4109) (2.9397, 9.3713) (2.8958, 9.3312) (2.8525, 9.2908) (2.8098, 9.25) (2.7678, 9.2089) (2.7265, 9.1673) (2.686, 9.1253) (2.6462, 9.0829) (2.6072, 9.0401) (2.5689, 8.997) (2.5313, 8.9535) (2.4944, 8.9097) (2.4582, 8.8655) (2.4228, 8.8209) (2.3882, 8.776) (2.3548, 8.7305) (2.3226, 8.6846) (2.2916, 8.6382) (2.2617, 8.5913) (2.2327, 8.544) (2.2044, 8.4966) (2.1766, 8.4489) (2.1496, 8.401) (2.1241, 8.3526) (2.101, 8.3034) (2.0852, 8.2631) (2.0753, 8.2322) (2.0696, 8.2113) (2.0669, 8.2008) knots -1 -1 -1 -1 -1 -1 -0.98571429 -0.97142857 -0.95714286 -0.94285714 -0.92857143 -0.91428571 -0.9 -0.88571429 -0.87142857 -0.85714286 -0.84285714 -0.82857143 -0.81428571 -0.8 -0.78571429 -0.77142857 -0.75714286 -0.74285714 -0.72857143 -0.71428571 -0.7 -0.68571429 -0.67142857 -0.65714286 -0.64285714 -0.62857143 -0.61428571 -0.6 -0.58571429 -0.57142857 -0.55714286 -0.54285714 -0.52857143 -0.51428571 -0.5 -0.48571429 -0.47142857 -0.45714286 -0.44285714 -0.42857143 -0.41428571 -0.4 -0.38571429 -0.37142857 -0.35714286 -0.34285714 -0.32857143 -0.31428571 -0.3 -0.28571429 -0.27142857 -0.25714286 -0.24285714 -0.22857143 -0.21428571 -0.2 -0.18571429 -0.17142857 -0.15714286 -0.14285714 -0.12857143 -0.11428571 -0.1 -0.08571429 -0.07142857 -0.05714286 -0.04285714 -0.02857143 -0.01428571 0 0 0 0 0 0
  arc A25 (0.5142, 5.505) -> (-0.5142, 5.505) centre (0, 0) ccw
  spline S10 degree 5 poles (-2.0669, 8.2008) (-2.0696, 8.2113) (-2.0753, 8.2322) (-2.0852, 8.2631) (-2.101, 8.3034) (-2.1241, 8.3526) (-2.1496, 8.401) (-2.1766, 8.4489) (-2.2044, 8.4966) (-2.2327, 8.544) (-2.2617, 8.5913) (-2.2916, 8.6382) (-2.3226, 8.6846) (-2.3548, 8.7305) (-2.3882, 8.776) (-2.4228, 8.8209) (-2.4582, 8.8655) (-2.4944, 8.9097) (-2.5313, 8.9535) (-2.5689, 8.997) (-2.6072, 9.0401) (-2.6462, 9.0829) (-2.686, 9.1253) (-2.7265, 9.1673) (-2.7678, 9.2089) (-2.8098, 9.25) (-2.8525, 9.2908) (-2.8958, 9.3312) (-2.9397, 9.3713) (-2.9842, 9.4109) (-3.0293, 9.4502) (-3.0751, 9.4891) (-3.1214, 9.5276) (-3.1684, 9.5657) (-3.2159, 9.6034) (-3.264, 9.6407) (-3.3127, 9.6776) (-3.3619, 9.7141) (-3.4117, 9.7502) (-3.462, 9.7859) (-3.5128, 9.8212) (-3.5641, 9.8561) (-3.616, 9.8906) (-3.6684, 9.9247) (-3.7212, 9.9584) (-3.7746, 9.9916) (-3.8284, 10.0245) (-3.8827, 10.0569) (-3.9375, 10.0889) (-3.9928, 10.1205) (-4.0485, 10.1517) (-4.1047, 10.1824) (-4.1613, 10.2127) (-4.2183, 10.2426) (-4.2758, 10.2721) (-4.3338, 10.3011) (-4.3921, 10.3297) (-4.4509, 10.3578) (-4.5101, 10.3856) (-4.5696, 10.4129) (-4.6296, 10.4397) (-4.69, 10.4661) (-4.7508, 10.4921) (-4.812, 10.5176) (-4.8735, 10.5427) (-4.9354, 10.5673) (-4.9977, 10.5915) (-5.0604, 10.6152) (-5.1234, 10.6384) (-5.1868, 10.6612) (-5.2505, 10.6836) (-5.3018, 10.7011) (-5.3404, 10.7141) (-5.3662, 10.7226) (-5.3791, 10.7268) knots 0 0 0 0 0 0 0.01428571 0.02857143 0.04285714 0.05714286 0.07142857 0.08571429 0.1 0.11428571 0.12857143 0.14285714 0.15714286 0.17142857 0.18571429 0.2 0.21428571 0.22857143 0.24285714 0.25714286 0.27142857 0.28571429 0.3 0.31428571 0.32857143 0.34285714 0.35714286 0.37142857 0.38571429 0.4 0.41428571 0.42857143 0.44285714 0.45714286 0.47142857 0.48571429 0.5 0.51428571 0.52857143 0.54285714 0.55714286 0.57142857 0.58571429 0.6 0.61428571 0.62857143 0.64285714 0.65714286 0.67142857 0.68571429 0.7 0.71428571 0.72857143 0.74285714 0.75714286 0.77142857 0.78571429 0.8 0.81428571 0.82857143 0.84285714 0.85714286 0.87142857 0.88571429 0.9 0.91428571 0.92857143 0.94285714 0.95714286 0.97142857 0.98571429 1 1 1 1 1 1
  arc A26 (-5.3791, 10.7268) -> (-6.6001, 10.0219) centre (0, 0) ccw
  spline S11 degree 5 poles (-6.6001, 10.0219) (-6.6029, 10.0086) (-6.6084, 9.9819) (-6.6165, 9.942) (-6.627, 9.8889) (-6.6395, 9.8225) (-6.6514, 9.7562) (-6.6628, 9.69) (-6.6736, 9.6239) (-6.6838, 9.5579) (-6.6935, 9.4919) (-6.7025, 9.4261) (-6.711, 9.3604) (-6.7189, 9.2947) (-6.7262, 9.2292) (-6.733, 9.1639) (-6.7391, 9.0986) (-6.7447, 9.0335) (-6.7497, 8.9685) (-6.7541, 8.9037) (-6.758, 8.839) (-6.7612, 8.7745) (-6.7638, 8.7101) (-6.7659, 8.6459) (-6.7674, 8.5819) (-6.7682, 8.5181) (-6.7685, 8.4545) (-6.7682, 8.391) (-6.7672, 8.3277) (-6.7657, 8.2647) (-6.7636, 8.2019) (-6.7609, 8.1392) (-6.7575, 8.0769) (-6.7536, 8.0147) (-6.749, 7.9528) (-6.7439, 7.8911) (-6.7381, 7.8297) (-6.7317, 7.7686) (-6.7247, 7.7077) (-6.7171, 7.6471) (-6.7088, 7.5868) (-6.6999, 7.5268) (-6.6904, 7.467) (-6.6803, 7.4077) (-6.6695, 7.3486) (-6.658, 7.2899) (-6.6459, 7.2315) (-6.6332, 7.1734) (-6.6199, 7.1157) (-6.6059, 7.0584) (-6.5912, 7.0014) (-6.5758, 6.9449) (-6.5597, 6.8888) (-6.5429, 6.8332) (-6.5254, 6.778) (-6.5072, 6.7233) (-6.4883, 6.669) (-6.4688, 6.6151) (-6.4486, 6.5616) (-6.4278, 6.5086) (-6.4061, 6.4563) (-6.3835, 6.4046) (-6.3598, 6.3537) (-6.3351, 6.3037) (-6.3094, 6.2544) (-6.283, 6.2056) (-6.2561, 6.1573) (-6.2287, 6.1095) (-6.2007, 6.0621) (-6.1715, 6.0158) (-6.1405, 5.9712) (-6.1134, 5.9374) (-6.0916, 5.9134) (-6.0764, 5.8979) (-6.0686, 5.8904) knots -1 -1 -1 -1 -1 -1 -0.98571429 -0.97142857 -0.95714286 -0.94285714 -0.92857143 -0.91428571 -0.9 -0.88571429 -0.87142857 -0.85714286 -0.84285714 -0.82857143 -0.81428571 -0.8 -0.78571429 -0.77142857 -0.75714286 -0.74285714 -0.72857143 -0.71428571 -0.7 -0.68571429 -0.67142857 -0.65714286 -0.64285714 -0.62857143 -0.61428571 -0.6 -0.58571429 -0.57142857 -0.55714286 -0.54285714 -0.52857143 -0.51428571 -0.5 -0.48571429 -0.47142857 -0.45714286 -0.44285714 -0.42857143 -0.41428571 -0.4 -0.38571429 -0.37142857 -0.35714286 -0.34285714 -0.32857143 -0.31428571 -0.3 -0.28571429 -0.27142857 -0.25714286 -0.24285714 -0.22857143 -0.21428571 -0.2 -0.18571429 -0.17142857 -0.15714286 -0.14285714 -0.12857143 -0.11428571 -0.1 -0.08571429 -0.07142857 -0.05714286 -0.04285714 -0.02857143 -0.01428571 0 0 0 0 0 0
  dimension "d9" = 7
  dimension "d10" = 10
  constraint concentric A0 A4
  constraint concentric A4 A5
  measures "d9" diameter of A4
  measures "d10" diameter of A5
extrude "Extrude3" add sketch "Sketch4" along normal blind 3 separate body contours A5 makes body 2
sketch "Sketch5" plane through (0, 0, 10) normal (0, 0, 1) x (-1, 0, 0)
  circle A0 centre (0, 0) radius 3.5
  circle A1 centre (0, 0) radius 5
extrude "Extrude4" add sketch "Sketch5" along normal blind 3 separate body makes body 3
sketch "Sketch6" plane through (0, 0, 13) normal (0, 0, 1) x (-1, 0, 0)
  circle A0 centre (0, 0) radius 3.5
  circle A1 centre (0, 0) radius 5
  circle A2 centre (0, 0) radius 5
  circle A3 centre (0, 0) radius 1.6
  line L0 (0, -1.6) -> (0, 1.6) construction
  line L1 (0, -1.6) -> (0, -1.1) construction
  line L2 (0, -1.1) -> (-1.1619, -1.1)
  line L3 (0, -1.1) -> (1.1619, -1.1)
  dimension "d15" = 10
  dimension "d20" = 3.2
  dimension "d21" = 0.5
  constraint concentric A0 A2
  constraint concentric A0 A3
  constraint coincident A3 L0.start
  constraint coincident A3 L0.end
  constraint vertical L0
  constraint parallel L0 L1
  constraint coincident A3 L2.end
  constraint perpendicular L1 L2
  constraint coincident A3 L3.end
  constraint perpendicular L0 L3
  measures "d15" diameter of A2
  measures "d20" diameter of A3
  measures "d21" distance of L0.start L1.end
extrude "Extrude5" add sketch "Sketch6" along normal blind 3 separate body contours A0 | A1 A2 | A3 L2 L3 picked at (0, -1.4304) makes body 4
combine "Combine1" operation add target body 2 tool bodies 3 4
extrude "Extrude6" add 1 faces at (0.1246, 2.3953, 16) along direction (0, 0, 1) blind 5 on bodies 2 bodies 2
extrude "Extrude7" add 1 faces at (0.0872, 1.8967, 13) along direction (0, 0, -1) blind 1.5 on bodies 2 bodies 2